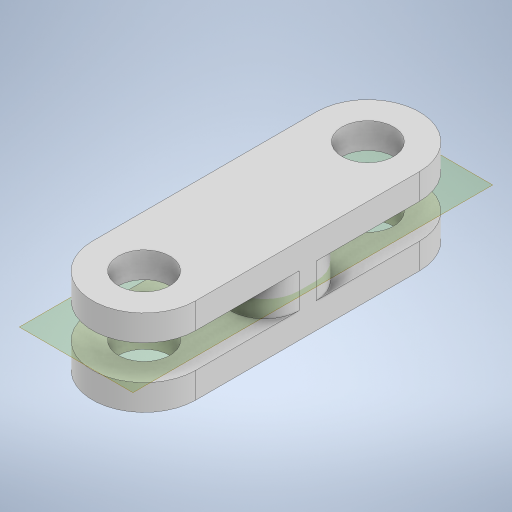
# Autodesk Inventor part: DAWN_chain_round
Saved by Autodesk Inventor 2024 (Build 280153000, 153)
## iProperties
Created: 2024-03-11
Part Number: DAWN_chain_round
Material: Generic
Document SubType Name: Modeling
Designer: magn1
Density: 1 g/cm^3
Appearance: Default
Author: magn1
Autodesk Inventor part; units mm, degrees
ref_plane "YZ Plane" through (0, 0, 0) normal (1, 0, 0) x (0, 1, 0)
ref_plane "XZ Plane" through (0, 0, 0) normal (0, 1, 0) x (-1, 0, 0)
ref_plane "XY Plane" through (0, 0, 0) normal (0, 0, 1) x (1, 0, 0)
sketch "Sketch1" plane through (0, 0, 0) normal (0, 1, 0) x (-1, 0, 0)
  line L0 (-3, 10) -> (3, 10)
  line L1 (3, 10) -> (3, -10)
  line L2 (3, -10) -> (-3, -10)
  line L3 (-3, -10) -> (-3, 10)
  line L4 (-3, 10) -> (3, -10) construction
  line L5 (3, 10) -> (-3, -10) construction
  line L6 (0, -10) -> (0, -6.5) construction
  line L7 (0, 10) -> (0, 6.5) construction
  circle A0 centre (0, 6.5) radius 1.5
  circle A1 centre (0, -6.5) radius 1.5
  point P0 (0, 0)
  dimension "d0" = 6
  dimension "d1" = 20
  dimension "d2" = 3.5
  dimension "d3" = 3.5
  dimension "d4" = 3
  dimension "d5" = 3
  constraints: 16 end point, 4 midpoint, 2 centre point, 2 coincident, 2 parallel, 2 vertical, 1 horizontal, 1 perpendicular
  measures "d0" distance of L1.end L2.end
  measures "d1" distance of L0.end L1.end
  measures "d2" distance of L6.start L6.end
  measures "d3" distance of L7.start L7.end
  measures "d4" diameter of A0
  measures "d5" diameter of A1
extrude "Extrusion1" add sketch "Sketch1" along normal blind 1.5
fillet "Fillet1" radius 2 4 edges at (3, 0.75, 10) (-3, 0.75, 10) (3, 0.75, -10) (-3, 0.75, -10)
sketch "Sketch2" plane through (0, 1.5, 0) normal (0, 1, 0) x (1, 0, 0)
  circle A0 centre (0, -6.5) radius 1.5 projected
  circle A1 centre (0, -6.5) radius 1.5
  circle A2 centre (0, -6.5) radius 3
  line L0 (-3, -6.5) -> (3, -6.5)
  line L1 (3, -6.5) -> (3, -10)
  line L2 (3, -10) -> (-3, -10)
  line L3 (-3, -10) -> (-3, -6.5)
  point P0 (0, 0)
  point P1 (3, -6.5)
  dimension "d9" = 6
  dimension "d10" = 3
  dimension "d11" = 3.5
  constraints: 8 end point, 2 coincident, 2 parallel, 2 vertical, 1 centre point, 1 horizontal, 1 perpendicular, 3 other
  measures "d10" diameter of A1
  measures "d11" distance between parallel lines of L2 L0
extrude "Extrusion2" cut sketch "Sketch2" against normal through all contours L1 L2 L3 A2
mirror "Mirror1" about plane through (0, 0, 0) normal (0, 0, 1) of "Extrusion2"
sketch "Sketch3" plane through (0, 1.5, 0) normal (0, 1, 0) x (1, 0, 0)
  line L0 (-3, 6.5) -> (-3, -6.5) projected
  line L1 (3, -2.5) -> (-3, -2.5)
  line L2 (-3, -2.5) -> (-3, 2.5)
  line L3 (-3, 2.5) -> (3, 2.5)
  line L4 (3, 2.5) -> (3, -2.5)
  line L5 (3, -2.5) -> (-3, 2.5) construction
  line L6 (-3, -2.5) -> (3, 2.5) construction
  point P0 (0, 0)
  dimension "d14" = 5
  constraints: 12 end point, 2 midpoint, 2 parallel, 1 horizontal, 1 perpendicular, 1 point on line
  measures "d14" distance of L1.end L2.end
extrude "Extrusion3" add sketch "Sketch3" along normal blind 2
ref_plane "Work Plane1" through (0, 2.5, 0) normal (0, -1, 0) x (1, 0, 0)
mirror "Mirror2" about plane through (0, 2.5, 0) normal (0, -1, 0) of "Extrusion1", "Fillet1", "Extrusion2", "Mirror1"
fillet "Fillet2" radius 2 4 edges at (3, 2.5, 2.5) (3, 2.5, -2.5) (-3, 2.5, 2.5) (-3, 2.5, -2.5)
body "Solid1"
